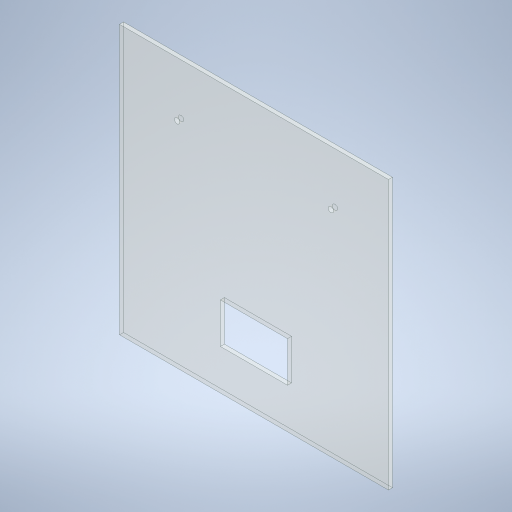
# Autodesk Inventor part: facef
Saved by Autodesk Inventor 2024 (Build 280153000, 153)
## iProperties
Created: 2023-06-07
Part Number: facef
Material: Glass
Document SubType Name: Modeling
Designer: shrus
Density: 2.18 g/cm^3
Appearance: Clear
Author: shrus
Autodesk Inventor part; units mm, degrees
ref_plane "YZ Plane" through (0, 0, 0) normal (1, 0, 0) x (0, 1, 0)
ref_plane "XZ Plane" through (0, 0, 0) normal (0, 1, 0) x (-1, 0, 0)
ref_plane "XY Plane" through (0, 0, 0) normal (0, 0, 1) x (1, 0, 0)
sketch "Sketch1" plane through (0, 0, 0) normal (0, 0, 1) x (1, 0, 0)
  line L0 (-12.121, 12.2642) -> (187.879, 12.2642)
  line L1 (187.879, 12.2642) -> (187.879, -187.7358)
  line L2 (187.879, -187.7358) -> (-12.121, -187.7358)
  line L3 (-12.121, -187.7358) -> (-12.121, 12.2642)
  point P0 (0, 0)
  dimension "d0" = 200
  dimension "d1" = 200
  dimension "d2" = 200
  constraints: 8 end point, 2 perpendicular, 1 horizontal
  measures "d0" distance of L0.start L0.end
  measures "d1" distance of L0.end L1.end
  measures "d2" distance of L1.end L2.end
extrude "Extrusion1" add sketch "Sketch1" along normal blind 3
sketch "Sketch2" plane through (0, 0, 3) normal (0, 0, 1) x (1, 0, 0)
  circle A0 centre (30.5932, -28.4894) radius 2.0324
  line L0 (187.879, -187.7358) -> (187.879, 12.2642) projected
  circle A1 centre (145.0597, -28.4894) radius 2.0324
  line L1 (62.879, -127.7358) -> (112.879, -127.7358)
  line L2 (112.879, -127.7358) -> (112.879, -157.7358)
  line L3 (112.879, -157.7358) -> (62.879, -157.7358)
  line L4 (62.879, -157.7358) -> (62.879, -127.7358)
  line L5 (-12.121, -187.7358) -> (187.879, -187.7358) projected
  line L6 (-12.121, 12.2642) -> (-12.121, -187.7358) projected
  point P0 (0, 0)
  point P1 (42.5932, -63.9945)
  point P2 (133.0597, -63.9945)
  point P3 (62.879, -142.7358)
  dimension "d14" = 12
  dimension "d15" = 12
  dimension "d16" = 50
  dimension "d17" = 30
  dimension "d18" = 30
  dimension "d19" = 75
  constraints: 8 end point, 2 centre point, 2 parallel, 1 coincident, 1 horizontal, 1 midpoint, 1 perpendicular
  measures "d14" horizontal distance of point (42.593, -63.994) A0.centre
  measures "d15" horizontal distance of point (145.06, -28.489) point (133.06, -63.994)
  measures "d16" distance of L2.end L3.end
  measures "d17" distance of L1.end L2.end
  measures "d18" distance between parallel lines of L5 L3
  measures "d19" distance from line of L6 point (62.879, -142.736)
extrude "Extrusion2" cut sketch "Sketch2" against normal blind 3
body "Solid1"
